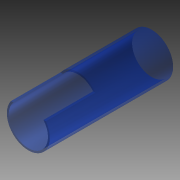
# Autodesk Inventor part: Main_Tubing_Al
Saved by Autodesk Inventor 2011 SP2 (Build 150309200, 309)
## iProperties
Created: 2012-03-18
Part Number: Main_Tubing_Al
Document SubType Name: Modeling
Designer: sungwook
Density: 1 g/cm^3
Author: sungwook
Autodesk Inventor part; units mm, degrees
ref_plane "YZ Plane" through (0, 0, 0) normal (1, 0, 0) x (0, 1, 0)
ref_plane "XY Plane" through (0, 0, 0) normal (0, 0, 1) x (1, 0, 0)
sketch "Sketch1" plane through (0, 0, 0) normal (0, 0, 1) x (1, 0, 0)
  circle A0 centre (0, 0) radius 14.2875
  circle A1 centre (0, 0) radius 13.0429
  dimension "d0" = 28.575
  dimension "d1" = 26.0858
  constraints: 2 centre point, 2 coincident
  measures "d0" diameter of A0
  measures "d1" diameter of A1
extrude "Extrusion1" add sketch "Sketch1" along normal blind 81.9912
ref_plane "POffset" through (0, 8.3, 0) normal (0, 1, 0) x (-1, 0, 0)
sketch "Sketch2" plane through (0, 8.3, 0) normal (0, 1, 0) x (-1, 0, 0)
  line L0 (11.6294, 81.9912) -> (11.6294, 0) projected
  line L1 (11.6294, 0) -> (10.0612, 0) projected
  line L2 (10.0612, 0) -> (10.0612, 81.9912) projected
  line L3 (10.0612, 81.9912) -> (11.6294, 81.9912) projected
  line L4 (-11.6294, 0) -> (-11.6294, 81.9912) projected
  line L5 (-11.6294, 81.9912) -> (-10.0612, 81.9912) projected
  line L6 (-10.0612, 81.9912) -> (-10.0612, 0) projected
  line L7 (-10.0612, 0) -> (-11.6294, 0) projected
  line L8 (-11.6294, 81.9912) -> (11.6294, 81.9912)
  line L9 (11.6294, 81.9912) -> (11.6294, 48.9912)
  line L10 (11.6294, 48.9912) -> (-11.6294, 48.9912)
  line L11 (-11.6294, 48.9912) -> (-11.6294, 81.9912)
  point P0 (0, 0)
  dimension "d5" = 33
  constraints: 8 end point, 2 parallel, 1 horizontal, 1 perpendicular, 1 point on line
  measures "d5" distance of L9.end L8.end
extrude "Extrusion2" cut sketch "Sketch2" along normal through all contours L0 L10 L2 L3 | L2 L10 L6 L8 | L6 L10 L4 L5
equation "\"d5\" = length"
equation "\"POffset\" = 8.3"
equation "\"d4\" = POffset"
equation "\"length\" = 33"
body "Solid1"
